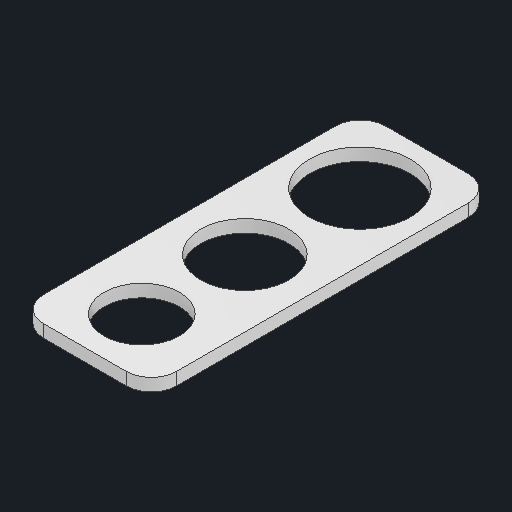
# Autodesk Inventor part: baicPart
Saved by Autodesk Inventor 2025.2 (Build 292293000, 293)
## iProperties
Company: FC-TORQUE
Created: 2025-03-14
Part Number: baicPart
Material: アルミニウム
Document SubType Name: Modeling
Designer: Keito Tamura
Density: 2.7 g/cm^3
Appearance: サテン
Mass: 379.336 g
Surface Area: 665.248 cm^2
Volume: 140.495 cm^3
Author: Keito Tamura
Autodesk Inventor part; units mm, degrees
ref_plane "YZ Plane" through (0, 0, 0) normal (1, 0, 0) x (0, 1, 0)
ref_plane "XZ Plane" through (0, 0, 0) normal (0, 1, 0) x (-1, 0, 0)
ref_plane "XY Plane" through (0, 0, 0) normal (0, 0, 1) x (1, 0, 0)
sketch "スケッチ2" plane through (0, 0, 0) normal (0, 1, 0) x (-1, 0, 0)
  circle A0 centre (0, 0) radius 3
  circle A1 centre (0, -8.1847) radius 3.5
  circle A2 centre (0, -17.3163) radius 4
  line L0 (3.2403, 4.5528) -> (-3.323, 4.5528)
  line L1 (-5.323, 2.5528) -> (-5.323, -20.6084)
  line L2 (-3.323, -22.6084) -> (3.2403, -22.6084)
  line L3 (5.2403, -20.6084) -> (5.2403, 2.5528)
  arc A3 (3.2403, -22.6084) -> (5.2403, -20.6084) centre (3.2403, -20.6084) ccw
  arc A4 (-5.323, -20.6084) -> (-3.323, -22.6084) centre (-3.323, -20.6084) ccw
  arc A5 (5.2403, 2.5528) -> (3.2403, 4.5528) centre (3.2403, 2.5528) ccw
  arc A6 (-3.323, 4.5528) -> (-5.323, 2.5528) centre (-3.323, 2.5528) ccw
  dimension "d34" = 6
  dimension "d35" = 7
  dimension "d36" = 8
  dimension "d37" = 2
  constraints: 8 end point, 8 point on circle, 8 tangent, 7 centre point, 3 equal radius, 2 parallel, 1 coincident, 1 horizontal, 1 perpendicular
  measures "d34" diameter of A0
  measures "d35" diameter of A1
  measures "d36" diameter of A2
  measures "d37" radius of A3
extrude "押し出し3" add sketch "スケッチ2" along normal blind 1
